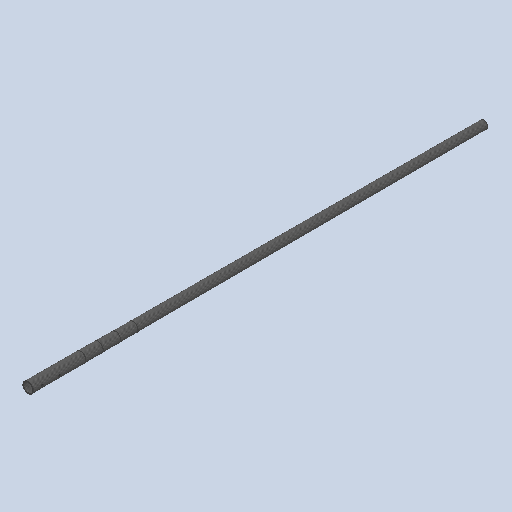
# Autodesk Inventor part: MAIN WING SPAR FINAL VERSION
Saved by Autodesk Inventor 2025.1 (Build 291241000, 241)
## iProperties
Category: <PART CATAGORY>
Created: 2024-10-31
Part Number: MAIN WING SPAR FINAL VERSION
Material: CFRP
Document SubType Name: Modeling
Designer: ex23650
Density: 1.43 g/cm^3
Appearance: Carbon Fiber
Title: <TITLE>
Author: ex23650
Revision Number: 1
Autodesk Inventor part; units mm, degrees
ref_plane "YZ Plane" through (0, 0, 0) normal (1, 0, 0) x (0, 1, 0)
ref_plane "XZ Plane" through (0, 0, 0) normal (0, 1, 0) x (-1, 0, 0)
ref_plane "XY Plane" through (0, 0, 0) normal (0, 0, 1) x (1, 0, 0)
sketch "Sketch6" plane through (0, 0, 0) normal (1, 0, 0) x (0, 1, 0)
  line L0 (0, 0) -> (13.55, 0) construction
  line L1 (0, 0) -> (1300, 0) construction
  line L2 (10.793, -1300) -> (13.55, 0)
  line L3 (13.55, 0) -> (14, 0)
  line L4 (13.55, 0) -> (14, 0) construction
  line L5 (10.793, -1300) -> (11.243, -1300)
  line L6 (10.793, -1300) -> (11.243, -1300) construction
  line L7 (11.243, -1300) -> (14, 0)
  line L8 (14, 0) -> (14.3, 0)
  line L9 (14, 0) -> (14.3, 0) construction
  line L10 (11.243, -1300) -> (11.543, -1300)
  line L11 (11.243, -1300) -> (11.543, -1300) construction
  line L12 (11.543, -1300) -> (14.3, 0)
  line L13 (0, 0) -> (300, 0) construction
  line L14 (13.6638, -300) -> (13.8138, -300)
  line L15 (14.3, 0) -> (14.45, 0)
  line L16 (14.3, 0) -> (14.45, 0) construction
  line L17 (14.45, 0) -> (13.8138, -300)
  line L18 (14.45, 0) -> (14.75, 0)
  line L19 (14.45, 0) -> (14.75, 0) construction
  line L20 (0, 0) -> (250, 0) construction
  line L21 (13.9198, -250) -> (14.2198, -250)
  line L22 (13.9198, -250) -> (14.2198, -250) construction
  line L23 (14.2198, -250) -> (14.75, 0)
  line L24 (14.75, 0) -> (15.05, 0)
  line L25 (14.75, 0) -> (15.05, 0) construction
  line L26 (0, 0) -> (200, 0) construction
  line L27 (14.3258, -200) -> (14.6258, -200)
  line L28 (14.3258, -200) -> (14.6258, -200) construction
  line L29 (14.6258, -200) -> (15.05, 0)
  line L30 (15.05, 0) -> (15.35, 0)
  line L31 (15.05, 0) -> (15.35, 0) construction
  line L32 (0, 0) -> (150, 0) construction
  line L33 (14.7319, -150) -> (15.0319, -150)
  line L34 (14.7319, -150) -> (15.0319, -150) construction
  line L35 (15.0319, -150) -> (15.35, 0)
  line L36 (0, 0) -> (0, -50)
  line L37 (0, 0) -> (50, 0) construction
  dimension "d91" = 0.45
  dimension "d93" = 0.45
  dimension "d94" = 0
  dimension "d95" = 0.3
  dimension "d96" = 0
  dimension "d97" = 0.3
  dimension "d98" = 0
  dimension "d102" = 0.15
  dimension "d104" = 0.15
  dimension "d105" = 0
  dimension "d106" = 0.3
  dimension "d107" = 0
  dimension "d111" = 0.3
  dimension "d112" = 0
  dimension "d113" = 0.3
  dimension "d114" = 0
  dimension "d118" = 0.3
  dimension "d119" = 0
  dimension "d120" = 0.3
  dimension "d121" = 0
  dimension "d125" = 0.3
  dimension "d126" = 0
  dimension "d127" = 50
  dimension "d128" = 90
  constraints: 76 end point, 21 horizontal, 12 equal length, 6 collinear, 3 point on line, 1 parallel, 1 perpendicular
  measures "d91" distance of L0.end L3.end
  measures "d93" distance of L2.start L5.end
  measures "d94" distance between parallel lines of L5 L6
  measures "d95" distance of L4.end L8.end
  measures "d96" distance between parallel lines of L8 L9
  measures "d97" distance of L6.end L10.end
  measures "d98" distance between parallel lines of L10 L11
  measures "d102" distance of L14.start L14.end
  measures "d104" distance of L9.end L15.end
  measures "d105" distance between parallel lines of L15 L16
  measures "d106" distance of L16.end L18.end
  measures "d107" distance between parallel lines of L18 L19
  measures "d111" distance of L21.start L21.end
  measures "d112" distance between parallel lines of L21 L22
  measures "d113" distance of L19.end L24.end
  measures "d114" distance between parallel lines of L24 L25
  measures "d118" distance of L27.start L27.end
  measures "d119" distance between parallel lines of L27 L28
  measures "d120" distance of L25.end L30.end
  measures "d121" distance between parallel lines of L30 L31
  measures "d125" distance of L33.start L33.end
  measures "d126" distance between parallel lines of L33 L34
  measures "d127" distance of L0.start L36.end
  measures "d128" angle of L36 L37
sketch "Sketch8" plane through (0, 0, 0) normal (1, 0, 0) x (0, 1, 0)
  line L0 (0, 0) -> (0, -25)
  line L1 (0, 0) -> (25, 0) construction
  line L2 (0, -25) -> (0, -75)
  circle A0 centre (0, -25) radius 3
  circle A1 centre (0, -75) radius 3
  dimension "d154" = 25
  dimension "d155" = 90
  dimension "d156" = 50
  dimension "d157" = 180
  dimension "d159" = 6
  dimension "d160" = 6
  constraints: 6 end point, 2 centre point, 2 coincident, 1 collinear, 1 horizontal, 1 perpendicular, 1 vertical
  measures "d154" distance of L0.start L0.end
  measures "d155" angle of L0 L1
  measures "d156" distance of L0.end L2.end
  measures "d157" angle of L2 L0
  measures "d159" diameter of A0
  measures "d160" diameter of A1
revolve "Revolution2" add sketch "Sketch6" angle 360 about axis through (0, 0, 0) along (0, 0, -1)
hole "Hole6" at (0, 0, -25) at (0, 0, -75) direction (-1, 0, 0) diameter 6 end through all both
